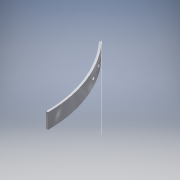
# Autodesk Inventor part: Part13
Saved by Autodesk Inventor 2016 (Build 200138000, 138)
## iProperties
Created: 2016-01-27
Part Number: Part13
Material: Aluminum 6061
Document SubType Name: Modeling
Designer: 278648
Density: 2.7 g/cm^3
Appearance: Aluminum - Flat
Mass: 36.017 g
Surface Area: 97.7111 cm^2
Volume: 13.3396 cm^3
User Status: in process
Author: 278648
Autodesk Inventor part; units mm, degrees
ref_plane "YZ Plane" through (0, 0, 0) normal (1, 0, 0) x (0, 1, 0)
ref_plane "XZ Plane" through (0, 0, 0) normal (0, 1, 0) x (-1, 0, 0)
ref_plane "XY Plane" through (0, 0, 0) normal (0, 0, 1) x (1, 0, 0)
sketch "Sketch1" plane through (0, 0, 0) normal (0, 1, 0) x (-1, 0, 0)
  arc A0 (-215.9, 0) -> (-152.6644, -152.6644) centre (0, 0) ccw
  arc A1 (-212.725, 0) -> (-150.4193, -150.4193) centre (0, 0) ccw
  line L0 (-150.4193, -150.4193) -> (-152.6644, -152.6644)
  line L1 (-212.725, 0) -> (-215.9, 0)
  dimension "d0" = 431.8
  dimension "d1" = 3.175
  dimension "d2" = 45
  constraints: 4 end point, 4 point on circle, 2 centre point, 2 coincident, 1 horizontal
  measures "d0" diameter of A0
  measures "d1" radial gap between concentric circles of A0 A1
  measures "d2" angle of L0 L1
extrude "Extrusion1" add sketch "Sketch1" along normal blind 25.4
ref_plane "Work Plane1" through (152.6644, 0, -152.6644) normal (0.7071, 0, -0.7071) x (0, 1, 0)
sketch "Sketch2" plane through (152.6644, 0, -152.6644) normal (0.7071, 0, -0.7071) x (0, 1, 0)
  circle A0 centre (12.7, 38.1) radius 3.3734
  line L0 (0, 0) -> (25.4, 0) projected
  circle A1 centre (12.7, 63.8969) radius 3.3734
  line L1 (25.4, 150.4193) -> (25.4, 0) projected
  dimension "d5" = 6.7469
  dimension "d6" = 38.1
  dimension "d7" = 6.7469
  dimension "d8" = 19.05
  dimension "d9" = 12.7
  dimension "d10" = 12.7
  constraints: 2 centre point
  measures "d5" diameter of A0
  measures "d6" distance from line of L0 A0.centre
  measures "d7" diameter of A1
  measures "d9" distance from line of L1 A1.centre
  measures "d10" distance from line of L1 A0.centre
extrude "Extrusion2" cut sketch "Sketch2" against normal blind 17.78
body "Solid1"
